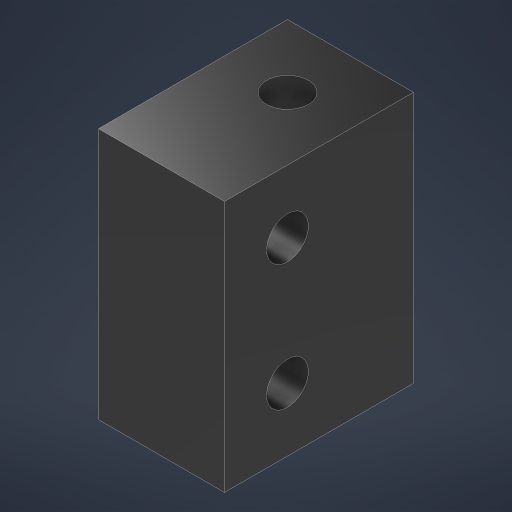
# Autodesk Inventor part: wing mount 1 v1
Saved by Autodesk Inventor 2024 (Build 280153000, 153)
## iProperties
Created: 2023-12-20
Part Number: wing mount 1 v1
Material: Generic
Document SubType Name: Modeling
Designer: elite
Density: 1 g/cm^3
Appearance: Glossy - Black
Author: elite
Autodesk Inventor part; units mm, degrees
ref_plane "YZ Plane" through (0, 0, 0) normal (1, 0, 0) x (0, 1, 0)
ref_plane "XZ Plane" through (0, 0, 0) normal (0, 1, 0) x (-1, 0, 0)
ref_plane "XY Plane" through (0, 0, 0) normal (0, 0, 1) x (1, 0, 0)
sketch "Sketch1" plane through (0, 0, 0) normal (1, 0, 0) x (0, 1, 0)
  line L0 (0, 0) -> (25.4, 0)
  line L1 (25.4, 0) -> (25.4, -19.05)
  line L2 (25.4, -19.05) -> (0, -19.05)
  line L3 (0, -19.05) -> (0, 0)
  line L4 (25.4, 0) -> (25.4, -6.35)
  line L5 (25.4, -6.35) -> (19.05, -6.35)
  line L6 (19.05, -6.35) -> (6.35, -6.35)
  circle A0 centre (19.05, -6.35) radius 2.1082
  circle A1 centre (6.35, -6.35) radius 2.1082
  dimension "d0" = 19.05
  dimension "d1" = 25.4
  dimension "d2" = 6.35
  dimension "d3" = 6.35
  dimension "d4" = 12.7
  dimension "d5" = 4.2164
  constraints: 14 end point, 2 centre point, 2 coincident, 2 parallel, 2 perpendicular, 2 point on line, 1 horizontal
  measures "d0" distance of L0.end L1.end
  measures "d1" distance of L1.end L2.end
  measures "d2" distance of L0.end L4.end
  measures "d3" distance of L4.end L5.end
  measures "d4" distance of L5.end L6.end
  measures "d5" diameter of A0
extrude "Extrusion1" add sketch "Sketch1" along normal blind 12.7
sketch "Sketch2" plane through (0, 25.4, 0) normal (0, 1, 0) x (1, 0, 0)
  line L0 (0, 0) -> (0, 19.05) projected
  line L1 (0, 19.05) -> (12.7, 19.05) projected
  line L2 (0, 19.05) -> (12.7, 19.05)
  line L3 (6.35, 19.05) -> (6.35, 12.7)
  circle A0 centre (6.35, 12.7) radius 2.1082
  dimension "d8" = 6.35
  dimension "d9" = 4.2164
  constraints: 4 end point, 1 centre point, 1 coincident, 1 collinear, 1 midpoint, 1 vertical
  measures "d8" distance of L3.start L3.end
  measures "d9" diameter of A0
extrude "Extrusion2" cut sketch "Sketch2" against normal blind 39.6875
body "Solid1"
